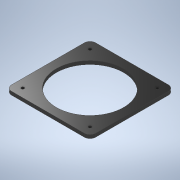
# Autodesk Inventor part: 150mm_Bearing_Plate
Saved by Autodesk Inventor 2020.4 (Build 244396010, 396A)
## iProperties
Created: 2021-09-01
Part Number: 150mm_Bearing_Plate
Material: ABS Plastic
Document SubType Name: Modeling
Designer: justi
Density: 1.06 g/cm^3
Appearance: Glossy - Black
Author: justi
Autodesk Inventor part; units mm, degrees
ref_plane "YZ Plane" through (0, 0, 0) normal (1, 0, 0) x (0, 1, 0)
ref_plane "XZ Plane" through (0, 0, 0) normal (0, 1, 0) x (-1, 0, 0)
ref_plane "XY Plane" through (0, 0, 0) normal (0, 0, 1) x (1, 0, 0)
sketch "Sketch1" plane through (0, 0, 0) normal (0, 1, 0) x (-1, 0, 0)
  line L0 (-75, 75) -> (75, 75)
  line L1 (75, 75) -> (75, -75)
  line L2 (75, -75) -> (-75, -75)
  line L3 (-75, -75) -> (-75, 75)
  line L4 (-75, 75) -> (75, -75) construction
  line L5 (75, 75) -> (-75, -75) construction
  circle A0 centre (0, 0) radius 60
  line L6 (-60, 60) -> (60, 60) construction
  line L7 (60, 60) -> (60, -60) construction
  line L8 (60, -60) -> (-60, -60) construction
  line L9 (-60, -60) -> (-60, 60) construction
  line L10 (-60, 60) -> (60, -60) construction
  line L11 (60, 60) -> (-60, -60) construction
  circle A1 centre (60, 60) radius 2.5
  circle A2 centre (60, -60) radius 2.5
  circle A3 centre (-60, 60) radius 2.5
  circle A4 centre (-60, -60) radius 2.5
  dimension "d0" = 150
  dimension "d1" = 150
  dimension "d2" = 120
  dimension "d3" = 120
  dimension "d4" = 5
  dimension "d5" = 5
  dimension "d6" = 5
  dimension "d7" = 5
  constraints: 24 end point, 5 centre point, 5 coincident, 4 midpoint, 4 parallel, 2 horizontal, 2 perpendicular, 1 point on line
  measures "d0" distance of L1.end L2.end
  measures "d1" distance of L0.end L1.end
  measures "d2" diameter of A0
  measures "d3" distance of L7.end L8.end
  measures "d4" diameter of A1
  measures "d5" diameter of A2
  measures "d6" diameter of A3
  measures "d7" diameter of A4
extrude "Extrusion1" add sketch "Sketch1" along normal blind 6
fillet "Fillet1" radius 10 4 edges at (-75, 3, 75) (75, 3, 75) (75, 3, -75) (-75, 3, -75)
body "Solid1"
